Autodesk Inventor part; units mm, degrees
(part 7 of 12)
  line L5353 (-7.555, 11.914) -> (-8.955, 11.914)
  line L5354 (-6.6345, 10.414) -> (-6.5735, 10.414)
  line L5355 (-7.304, 11.914) -> (-7.304, 8.914)
  line L5356 (-7.304, 8.914) -> (-5.904, 8.914)
  line L5357 (-5.904, 8.914) -> (-5.904, 11.914)
  line L5358 (-5.904, 11.914) -> (-7.304, 11.914)
  line L5359 (-10.1295, 25.019) -> (-10.1905, 25.019)
  line L5360 (-9.46, 23.519) -> (-9.46, 26.519)
  line L5361 (-9.46, 26.519) -> (-10.86, 26.519)
  line L5362 (-10.86, 26.519) -> (-10.86, 23.519)
  line L5363 (-10.86, 23.519) -> (-9.46, 23.519)
  line L5364 (-12.065, 6.4465) -> (-12.065, 6.5075)
  line L5365 (-13.565, 5.777) -> (-10.565, 5.777)
  line L5366 (-10.565, 5.777) -> (-10.565, 7.177)
  line L5367 (-10.565, 7.177) -> (-13.565, 7.177)
  line L5368 (-13.565, 7.177) -> (-13.565, 5.777)
  line L5369 (-25.5575, 7.747) -> (-25.4965, 7.747)
  line L5370 (-26.227, 9.247) -> (-26.227, 6.247)
  line L5371 (-26.227, 6.247) -> (-24.827, 6.247)
  line L5372 (-24.827, 6.247) -> (-24.827, 9.247)
  line L5373 (-24.827, 9.247) -> (-26.227, 9.247)
  line L5374 (-25.4965, 25.019) -> (-25.5575, 25.019)
  line L5375 (-24.827, 23.519) -> (-24.827, 26.519)
  line L5376 (-24.827, 26.519) -> (-26.227, 26.519)
  line L5377 (-26.227, 26.519) -> (-26.227, 23.519)
  line L5378 (-26.227, 23.519) -> (-24.827, 23.519)
  line L5379 (-28.8595, 26.797) -> (-28.7985, 26.797)
  line L5380 (-29.529, 28.297) -> (-29.529, 25.297)
  line L5381 (-29.529, 25.297) -> (-28.129, 25.297)
  line L5382 (-28.129, 25.297) -> (-28.129, 28.297)
  line L5383 (-28.129, 28.297) -> (-29.529, 28.297)
  line L5384 (-6.928, 26.273) -> (-6.928, 27.773)
  line L5385 (-6.928, 27.773) -> (-9.328, 27.773)
  line L5386 (-9.328, 27.773) -> (-9.328, 26.273)
  line L5387 (-6.928, 24.273) -> (-6.928, 23.173)
  line L5388 (-6.928, 23.173) -> (-7.328, 22.773)
  line L5389 (-7.328, 22.773) -> (-8.928, 22.773)
  line L5390 (-8.928, 22.773) -> (-9.328, 23.173)
  line L5391 (-9.328, 23.173) -> (-9.328, 24.273)
  line L5392 (-9.144, 24.892) -> (-7.112, 24.892)
  line L5393 (-22.971, 41.967) -> (-24.471, 41.967)
  line L5394 (-24.471, 41.967) -> (-24.471, 39.567)
  line L5395 (-24.471, 39.567) -> (-22.971, 39.567)
  line L5396 (-20.971, 41.967) -> (-19.871, 41.967)
  line L5397 (-19.871, 41.967) -> (-19.471, 41.567)
  line L5398 (-19.471, 41.567) -> (-19.471, 39.967)
  line L5399 (-19.471, 39.967) -> (-19.871, 39.567)
  line L5400 (-19.871, 39.567) -> (-20.971, 39.567)
  line L5401 (-21.59, 39.751) -> (-21.59, 41.783)
  line L5402 (-8.2245, 19.812) -> (-8.2855, 19.812)
  line L5403 (-7.555, 18.312) -> (-7.555, 21.312)
  line L5404 (-7.555, 21.312) -> (-8.955, 21.312)
  line L5405 (-8.955, 21.312) -> (-8.955, 18.312)
  line L5406 (-8.955, 18.312) -> (-7.555, 18.312)
  line L5407 (-17.673, 40.4695) -> (-17.673, 40.5305)
  line L5408 (-19.173, 39.8) -> (-16.173, 39.8)
  line L5409 (-16.173, 39.8) -> (-16.173, 41.2)
  line L5410 (-16.173, 41.2) -> (-19.173, 41.2)
  line L5411 (-19.173, 41.2) -> (-19.173, 39.8)
  line L5412 (-22.0305, 35.9) -> (-21.9695, 35.9)
  line L5413 (-22.7, 37.4) -> (-22.7, 34.4)
  line L5414 (-22.7, 34.4) -> (-21.3, 34.4)
  line L5415 (-21.3, 34.4) -> (-21.3, 37.4)
  line L5416 (-21.3, 37.4) -> (-22.7, 37.4)
  line L5417 (-19.3, 32.0695) -> (-19.3, 32.1305)
  line L5418 (-20.8, 31.4) -> (-17.8, 31.4)
  line L5419 (-17.8, 31.4) -> (-17.8, 32.8)
  line L5420 (-17.8, 32.8) -> (-20.8, 32.8)
  line L5421 (-20.8, 32.8) -> (-20.8, 31.4)
  line L5422 (-22.0305, 32.2) -> (-21.9695, 32.2)
  line L5423 (-22.7, 33.7) -> (-22.7, 30.7)
  line L5424 (-22.7, 30.7) -> (-21.3, 30.7)
  line L5425 (-21.3, 30.7) -> (-21.3, 33.7)
  line L5426 (-21.3, 33.7) -> (-22.7, 33.7)
  line L5427 (-13.7305, 37.6) -> (-13.6695, 37.6)
  line L5428 (-14.4, 39.1) -> (-14.4, 36.1)
  line L5429 (-14.4, 36.1) -> (-13, 36.1)
  line L5430 (-13, 36.1) -> (-13, 39.1)
  line L5431 (-13, 39.1) -> (-14.4, 39.1)
  line L5432 (-12.7, 36.2) -> (-11.3, 36.2)
  line L5433 (-11.3, 36.2) -> (-11.3, 39)
  line L5434 (-11.3, 39) -> (-12.7, 39)
  line L5435 (-12.7, 39) -> (-12.7, 36.2)
  line L5436 (-5.842, 14.0005) -> (-5.842, 13.9395)
  line L5437 (-4.342, 14.67) -> (-7.342, 14.67)
  line L5438 (-7.342, 14.67) -> (-7.342, 13.27)
  line L5439 (-7.342, 13.27) -> (-4.342, 13.27)
  line L5440 (-4.342, 13.27) -> (-4.342, 14.67)
  line L5441 (-5.842, 19.5275) -> (-5.842, 19.5885)
  line L5442 (-7.342, 18.858) -> (-4.342, 18.858)
  line L5443 (-4.342, 18.858) -> (-4.342, 20.258)
  line L5444 (-4.342, 20.258) -> (-7.342, 20.258)
  line L5445 (-7.342, 20.258) -> (-7.342, 18.858)
  line L5446 (-29.3586, 19.8336) -> (-29.3154, 19.7904)
  line L5447 (-28.7713, 21.3676) -> (-30.8926, 19.2463)
  line L5448 (-30.8926, 19.2463) -> (-29.9027, 18.2564)
  line L5449 (-29.9027, 18.2564) -> (-27.7814, 20.3777)
  line L5450 (-27.7814, 20.3777) -> (-28.7713, 21.3676)
  line L5451 (-19.685, 6.4465) -> (-19.685, 6.5075)
  line L5452 (-21.185, 5.777) -> (-18.185, 5.777)
  line L5453 (-18.185, 5.777) -> (-18.185, 7.177)
  line L5454 (-18.185, 7.177) -> (-21.185, 7.177)
  line L5455 (-21.185, 7.177) -> (-21.185, 5.777)
  line L5456 (-18.0086, 3.2766) -> (-18.0086, 4.0894)
  line L5457 (-18.0086, 4.0894) -> (-18.5674, 4.0894)
  line L5458 (-20.8534, 4.0894) -> (-20.8534, 3.2766)
  line L5459 (-20.2946, 4.0894) -> (-20.8534, 4.0894)
  line L5460 (-0.381, 41.148) -> (-0.635, 41.148)
  line L5461 (-5.969, 41.148) -> (-6.223, 41.148)
  circle A419 centre (-3.302, 41.148) radius 2.921
  circle A420 centre (-3.302, 41.148) radius 1.5
  line L5462 (-35.179, 41.148) -> (-34.925, 41.148)
  line L5463 (-29.591, 41.148) -> (-29.337, 41.148)
  circle A421 centre (-32.258, 41.148) radius 2.921
  circle A422 centre (-32.258, 41.148) radius 1.5
  line L5464 (-35.179, 4.699) -> (-35.179, 3.429)
  line L5465 (-35.179, 3.429) -> (-34.544, 2.794)
  line L5466 (-34.544, 2.794) -> (-33.274, 2.794)
  line L5467 (-33.274, 2.794) -> (-32.639, 3.429)
  line L5468 (-34.544, 7.874) -> (-35.179, 7.239)
  line L5469 (-35.179, 7.239) -> (-35.179, 5.969)
  line L5470 (-35.179, 5.969) -> (-34.544, 5.334)
  line L5471 (-34.544, 5.334) -> (-33.274, 5.334)
  line L5472 (-33.274, 5.334) -> (-32.639, 5.969)
  line L5473 (-32.639, 5.969) -> (-32.639, 7.239)
  line L5474 (-32.639, 7.239) -> (-33.274, 7.874)
  line L5475 (-35.179, 4.699) -> (-34.544, 5.334)
  line L5476 (-33.274, 5.334) -> (-32.639, 4.699)
  line L5477 (-32.639, 3.429) -> (-32.639, 4.699)
  line L5478 (-35.179, 12.319) -> (-35.179, 11.049)
  line L5479 (-35.179, 11.049) -> (-34.544, 10.414)
  line L5480 (-34.544, 10.414) -> (-33.274, 10.414)
  line L5481 (-33.274, 10.414) -> (-32.639, 11.049)
  line L5482 (-34.544, 10.414) -> (-35.179, 9.779)
  line L5483 (-35.179, 9.779) -> (-35.179, 8.509)
  line L5484 (-35.179, 8.509) -> (-34.544, 7.874)
  line L5485 (-34.544, 7.874) -> (-33.274, 7.874)
  line L5486 (-33.274, 7.874) -> (-32.639, 8.509)
  line L5487 (-32.639, 8.509) -> (-32.639, 9.779)
  line L5488 (-32.639, 9.779) -> (-33.274, 10.414)
  line L5489 (-34.544, 15.494) -> (-35.179, 14.859)
  line L5490 (-35.179, 14.859) -> (-35.179, 13.589)
  line L5491 (-35.179, 13.589) -> (-34.544, 12.954)
  line L5492 (-34.544, 12.954) -> (-33.274, 12.954)
  line L5493 (-33.274, 12.954) -> (-32.639, 13.589)
  line L5494 (-32.639, 13.589) -> (-32.639, 14.859)
  line L5495 (-32.639, 14.859) -> (-33.274, 15.494)
  line L5496 (-35.179, 12.319) -> (-34.544, 12.954)
  line L5497 (-33.274, 12.954) -> (-32.639, 12.319)
  line L5498 (-32.639, 11.049) -> (-32.639, 12.319)
  line L5499 (-35.179, 19.939) -> (-35.179, 18.669)
  line L5500 (-35.179, 18.669) -> (-34.544, 18.034)
  line L5501 (-34.544, 18.034) -> (-33.274, 18.034)
  line L5502 (-33.274, 18.034) -> (-32.639, 18.669)
  line L5503 (-34.544, 18.034) -> (-35.179, 17.399)
  line L5504 (-35.179, 17.399) -> (-35.179, 16.129)
  line L5505 (-35.179, 16.129) -> (-34.544, 15.494)
  line L5506 (-34.544, 15.494) -> (-33.274, 15.494)
  line L5507 (-33.274, 15.494) -> (-32.639, 16.129)
  line L5508 (-32.639, 16.129) -> (-32.639, 17.399)
  line L5509 (-32.639, 17.399) -> (-33.274, 18.034)
  line L5510 (-34.544, 20.574) -> (-33.274, 20.574)
  line L5511 (-35.179, 19.939) -> (-34.544, 20.574)
  line L5512 (-33.274, 20.574) -> (-32.639, 19.939)
  line L5513 (-32.639, 18.669) -> (-32.639, 19.939)
  line L5514 (-35.179, 2.159) -> (-35.179, 0.889)
  line L5515 (-35.179, 0.889) -> (-34.544, 0.254)
  line L5516 (-34.544, 0.254) -> (-33.274, 0.254)
  line L5517 (-33.274, 0.254) -> (-32.639, 0.889)
  line L5518 (-35.179, 2.159) -> (-34.544, 2.794)
  line L5519 (-33.274, 2.794) -> (-32.639, 2.159)
  line L5520 (-32.639, 0.889) -> (-32.639, 2.159)
  line L5521 (-2.921, 4.699) -> (-2.921, 3.429)
  line L5522 (-2.921, 3.429) -> (-2.286, 2.794)
  line L5523 (-2.286, 2.794) -> (-1.016, 2.794)
  line L5524 (-1.016, 2.794) -> (-0.381, 3.429)
  line L5525 (-2.286, 7.874) -> (-2.921, 7.239)
  line L5526 (-2.921, 7.239) -> (-2.921, 5.969)
  line L5527 (-2.921, 5.969) -> (-2.286, 5.334)
  line L5528 (-2.286, 5.334) -> (-1.016, 5.334)
  line L5529 (-1.016, 5.334) -> (-0.381, 5.969)
  line L5530 (-0.381, 5.969) -> (-0.381, 7.239)
  line L5531 (-0.381, 7.239) -> (-1.016, 7.874)
  line L5532 (-2.921, 4.699) -> (-2.286, 5.334)
  line L5533 (-1.016, 5.334) -> (-0.381, 4.699)
  line L5534 (-0.381, 3.429) -> (-0.381, 4.699)
  line L5535 (-2.921, 12.319) -> (-2.921, 11.049)
  line L5536 (-2.921, 11.049) -> (-2.286, 10.414)
  line L5537 (-2.286, 10.414) -> (-1.016, 10.414)
  line L5538 (-1.016, 10.414) -> (-0.381, 11.049)
  line L5539 (-2.286, 10.414) -> (-2.921, 9.779)
  line L5540 (-2.921, 9.779) -> (-2.921, 8.509)
  line L5541 (-2.921, 8.509) -> (-2.286, 7.874)
  line L5542 (-2.286, 7.874) -> (-1.016, 7.874)
  line L5543 (-1.016, 7.874) -> (-0.381, 8.509)
  line L5544 (-0.381, 8.509) -> (-0.381, 9.779)
  line L5545 (-0.381, 9.779) -> (-1.016, 10.414)
  line L5546 (-2.286, 15.494) -> (-2.921, 14.859)
  line L5547 (-2.921, 14.859) -> (-2.921, 13.589)
  line L5548 (-2.921, 13.589) -> (-2.286, 12.954)
  line L5549 (-2.286, 12.954) -> (-1.016, 12.954)
  line L5550 (-1.016, 12.954) -> (-0.381, 13.589)
  line L5551 (-0.381, 13.589) -> (-0.381, 14.859)
  line L5552 (-0.381, 14.859) -> (-1.016, 15.494)
  line L5553 (-2.921, 12.319) -> (-2.286, 12.954)
  line L5554 (-1.016, 12.954) -> (-0.381, 12.319)
  line L5555 (-0.381, 11.049) -> (-0.381, 12.319)
  line L5556 (-2.921, 19.939) -> (-2.921, 18.669)
  line L5557 (-2.921, 18.669) -> (-2.286, 18.034)
  line L5558 (-2.286, 18.034) -> (-1.016, 18.034)
  line L5559 (-1.016, 18.034) -> (-0.381, 18.669)
  line L5560 (-2.286, 18.034) -> (-2.921, 17.399)
  line L5561 (-2.921, 17.399) -> (-2.921, 16.129)
  line L5562 (-2.921, 16.129) -> (-2.286, 15.494)
  line L5563 (-2.286, 15.494) -> (-1.016, 15.494)
  line L5564 (-1.016, 15.494) -> (-0.381, 16.129)
  line L5565 (-0.381, 16.129) -> (-0.381, 17.399)
  line L5566 (-0.381, 17.399) -> (-1.016, 18.034)
  line L5567 (-2.286, 20.574) -> (-1.016, 20.574)
  line L5568 (-2.921, 19.939) -> (-2.286, 20.574)
  line L5569 (-1.016, 20.574) -> (-0.381, 19.939)
  line L5570 (-0.381, 18.669) -> (-0.381, 19.939)
  line L5571 (-2.921, 2.159) -> (-2.921, 0.889)
  line L5572 (-2.921, 0.889) -> (-2.286, 0.254)
  line L5573 (-2.286, 0.254) -> (-1.016, 0.254)
  line L5574 (-1.016, 0.254) -> (-0.381, 0.889)
  line L5575 (-2.921, 2.159) -> (-2.286, 2.794)
  line L5576 (-1.016, 2.794) -> (-0.381, 2.159)
  line L5577 (-0.381, 0.889) -> (-0.381, 2.159)
  line L5578 (-31.369, 9.779) -> (-31.369, 8.509)
  line L5579 (-31.369, 8.509) -> (-30.734, 7.874)
  line L5580 (-30.734, 7.874) -> (-29.464, 7.874)
  line L5581 (-29.464, 7.874) -> (-28.829, 8.509)
  line L5582 (-30.734, 12.954) -> (-31.369, 12.319)
  line L5583 (-31.369, 12.319) -> (-31.369, 11.049)
  line L5584 (-31.369, 11.049) -> (-30.734, 10.414)
  line L5585 (-30.734, 10.414) -> (-29.464, 10.414)
  line L5586 (-29.464, 10.414) -> (-28.829, 11.049)
  line L5587 (-28.829, 11.049) -> (-28.829, 12.319)
  line L5588 (-28.829, 12.319) -> (-29.464, 12.954)
  line L5589 (-31.369, 9.779) -> (-30.734, 10.414)
  line L5590 (-29.464, 10.414) -> (-28.829, 9.779)
  line L5591 (-28.829, 8.509) -> (-28.829, 9.779)
  line L5592 (-31.369, 17.399) -> (-31.369, 16.129)
  line L5593 (-31.369, 16.129) -> (-30.734, 15.494)
  line L5594 (-30.734, 15.494) -> (-29.464, 15.494)
  line L5595 (-29.464, 15.494) -> (-28.829, 16.129)
  line L5596 (-30.734, 15.494) -> (-31.369, 14.859)
  line L5597 (-31.369, 14.859) -> (-31.369, 13.589)
  line L5598 (-31.369, 13.589) -> (-30.734, 12.954)
  line L5599 (-30.734, 12.954) -> (-29.464, 12.954)
  line L5600 (-29.464, 12.954) -> (-28.829, 13.589)
  line L5601 (-28.829, 13.589) -> (-28.829, 14.859)
  line L5602 (-28.829, 14.859) -> (-29.464, 15.494)
  line L5603 (-30.734, 18.034) -> (-29.464, 18.034)
  line L5604 (-31.369, 17.399) -> (-30.734, 18.034)
  line L5605 (-29.464, 18.034) -> (-28.829, 17.399)
  line L5606 (-28.829, 16.129) -> (-28.829, 17.399)
  line L5607 (-31.369, 7.239) -> (-31.369, 5.969)
  line L5608 (-31.369, 5.969) -> (-30.734, 5.334)
  line L5609 (-30.734, 5.334) -> (-29.464, 5.334)
  line L5610 (-29.464, 5.334) -> (-28.829, 5.969)
  line L5611 (-31.369, 7.239) -> (-30.734, 7.874)
  line L5612 (-29.464, 7.874) -> (-28.829, 7.239)
  line L5613 (-28.829, 5.969) -> (-28.829, 7.239)
  line L5614 (-5.653, 11.914) -> (-5.653, 8.914)
  line L5615 (-5.653, 8.914) -> (-4.253, 8.914)
  line L5616 (-4.253, 8.914) -> (-4.253, 11.914)
  line L5617 (-4.253, 11.914) -> (-5.653, 11.914)
  line L5618 (-24.487, 5.777) -> (-21.487, 5.777)
  line L5619 (-21.487, 5.777) -> (-21.487, 7.177)
  line L5620 (-21.487, 7.177) -> (-24.487, 7.177)
  line L5621 (-24.487, 7.177) -> (-24.487, 5.777)
  line L5622 (-1.24, 31.399) -> (-0.94, 31.399)
  line L5623 (-0.94, 31.399) -> (-0.94, 28.799)
  line L5624 (-0.94, 28.799) -> (-1.24, 28.799)
  line L5625 (-3.84, 31.399) -> (-4.14, 31.399)
  line L5626 (-4.14, 31.399) -> (-4.14, 28.799)
  line L5627 (-4.14, 28.799) -> (-3.84, 28.799)
  line L5628 (-3.94, 31.899) -> (-3.94, 32.499)
  line L5629 (-3.94, 32.499) -> (-3.34, 32.499)
  line L5630 (-33.1614, 34.4142) -> (-33.5857, 33.9899)
  line L5631 (-33.5857, 33.9899) -> (-34.7171, 35.1213)
  line L5632 (-34.7171, 35.1213) -> (-34.2928, 35.5456)
  line L5633 (-31.7472, 35.8284) -> (-31.3229, 36.2527)
  line L5634 (-31.3229, 36.2527) -> (-32.4543, 37.3841)
  line L5635 (-32.4543, 37.3841) -> (-32.8786, 36.9598)
  line L5636 (-32.3129, 35.4042) -> (-32.8079, 35.8991)
  line L5637 (-32.8079, 35.8991) -> (-33.3028, 36.3941)
  line L5638 (-32.8079, 35.8991) -> (-32.8079, 35.0506)
  line L5639 (-32.8079, 35.0506) -> (-33.6564, 35.8991)
  line L5640 (-33.6564, 35.8991) -> (-32.8079, 35.8991)
  line L5641 (-3.8128, 35.8284) -> (-4.2371, 36.2527)
  line L5642 (-4.2371, 36.2527) -> (-3.1057, 37.3841)
  line L5643 (-3.1057, 37.3841) -> (-2.6814, 36.9598)
  line L5644 (-2.3986, 34.4142) -> (-1.9743, 33.9899)
  line L5645 (-1.9743, 33.9899) -> (-0.8429, 35.1213)
  line L5646 (-0.8429, 35.1213) -> (-1.2672, 35.5456)
  line L5647 (-2.8228, 34.9799) -> (-2.3279, 35.4749)
  line L5648 (-2.3279, 35.4749) -> (-1.8329, 35.9698)
  line L5649 (-2.3279, 35.4749) -> (-3.1764, 35.4749)
  line L5650 (-3.1764, 35.4749) -> (-2.3279, 36.3234)
  line L5651 (-2.3279, 36.3234) -> (-2.3279, 35.4749)
  line L5652 (-9.78, 28.068) -> (-9.78, 34.091)
  line L5653 (-9.78, 34.091) -> (-9.78, 38.045)
  line L5654 (-9.78, 38.045) -> (-9.78, 44.068)
  line L5655 (-9.78, 44.068) -> (-25.78, 44.068)
  line L5656 (-25.78, 44.068) -> (-25.78, 38.045)
  line L5657 (-25.78, 38.045) -> (-25.78, 34.091)
  line L5658 (-25.78, 34.091) -> (-25.78, 28.068)
  line L5659 (-25.78, 28.068) -> (-9.78, 28.068)
  arc A423 (-9.78, 34.091) -> (-9.78, 38.045) centre (-7.803, 36.068) ccw
  arc A424 (-25.78, 38.045) -> (-25.78, 34.091) centre (-27.757, 36.068) ccw
  line L5660 (-10.78, 29.068) -> (-24.78, 29.068)
  line L5661 (-24.78, 29.068) -> (-24.78, 43.068)
  line L5662 (-24.78, 43.068) -> (-10.78, 43.068)
  line L5663 (-10.78, 43.068) -> (-10.78, 29.068)
  line L5664 (-27.051, 40.005) -> (-26.67, 39.878)
  line L5665 (-26.67, 39.878) -> (-26.543, 40.005)
  line L5666 (-26.543, 40.005) -> (-26.797, 40.386)
  line L5667 (-26.797, 40.386) -> (-26.543, 40.767)
  line L5668 (-26.543, 40.767) -> (-26.289, 40.767)
  line L5669 (-26.289, 40.767) -> (-26.289, 41.021)
  line L5670 (-26.289, 41.021) -> (-26.67, 41.021)
  line L5671 (-26.67, 41.021) -> (-26.797, 41.402)
  line L5672 (-26.797, 41.402) -> (-26.543, 41.783)
  line L5673 (-26.543, 41.783) -> (-26.67, 41.91)
  line L5674 (-26.67, 41.91) -> (-27.051, 41.656)
  line L5675 (-27.051, 41.656) -> (-27.432, 41.91)
  line L5676 (-27.432, 41.91) -> (-27.432, 42.164)
  line L5677 (-27.432, 42.164) -> (-27.686, 42.164)
  line L5678 (-27.686, 42.164) -> (-27.813, 41.783)
  line L5679 (-27.813, 41.783) -> (-28.194, 41.656)
  line L5680 (-28.194, 41.656) -> (-28.448, 41.91)
  line L5681 (-28.448, 41.91) -> (-28.575, 41.783)
  line L5682 (-28.575, 41.783) -> (-28.448, 41.402)
  line L5683 (-28.448, 41.402) -> (-28.575, 41.021)
  line L5684 (-28.575, 41.021) -> (-28.956, 41.021)
  line L5685 (-28.956, 41.021) -> (-28.829, 40.767)
  line L5686 (-28.829, 40.767) -> (-28.448, 40.64)
  line L5687 (-28.448, 40.64) -> (-28.448, 40.259)
  line L5688 (-28.448, 40.259) -> (-28.575, 40.005)
  line L5689 (-28.575, 40.005) -> (-28.448, 39.878)
  line L5690 (-28.448, 39.878) -> (-28.194, 40.005)
  line L5691 (-28.194, 40.005) -> (-28.067, 40.005)
  line L5692 (-28.067, 40.005) -> (-27.94, 40.386)
  line L5693 (-27.94, 40.386) -> (-28.194, 40.894)
  line L5694 (-28.194, 40.894) -> (-27.94, 41.275)
  line L5695 (-27.94, 41.275) -> (-27.559, 41.402)
  line L5696 (-27.559, 41.402) -> (-27.178, 41.275)
  line L5697 (-27.178, 41.275) -> (-27.051, 40.894)
  line L5698 (-27.051, 40.894) -> (-27.178, 40.513)
  line L5699 (-27.178, 40.513) -> (-27.305, 40.386)
  line L5700 (-27.305, 40.386) -> (-27.051, 40.005)
  line L5701 (-26.6192, 39.9288) -> (-26.8224, 39.9288)
  line L5702 (-28.3464, 39.9288) -> (-28.4988, 39.9288)
  line L5703 (-26.5938, 40.0812) -> (-27.1018, 40.0812)
  line L5704 (-28.0416, 40.0812) -> (-28.5369, 40.0812)
  line L5705 (-26.6954, 40.2336) -> (-27.2034, 40.2336)
  line L5706 (-27.9908, 40.2336) -> (-28.4607, 40.2336)
  line L5707 (-26.797, 40.386) -> (-27.305, 40.386)
  line L5708 (-27.94, 40.386) -> (-28.448, 40.386)
  line L5709 (-26.6954, 40.5384) -> (-27.1695, 40.5384)
  line L5710 (-28.0162, 40.5384) -> (-28.448, 40.5384)
  line L5711 (-26.5938, 40.6908) -> (-27.1187, 40.6908)
  line L5712 (-28.0924, 40.6908) -> (-28.6004, 40.6908)
  line L5713 (-26.289, 40.8432) -> (-27.0679, 40.8432)
  line L5714 (-28.1686, 40.8432) -> (-28.8671, 40.8432)
  line L5715 (-26.289, 40.9956) -> (-27.0849, 40.9956)
  line L5716 (-28.1263, 40.9956) -> (-28.9433, 40.9956)
  line L5717 (-26.7123, 41.148) -> (-27.1357, 41.148)
  line L5718 (-28.0247, 41.148) -> (-28.5327, 41.148)
  line L5719 (-26.7631, 41.3004) -> (-27.2542, 41.3004)
  line L5720 (-27.8638, 41.3004) -> (-28.4819, 41.3004)
  line L5721 (-26.7631, 41.4528) -> (-28.4649, 41.4528)
  line L5722 (-26.6615, 41.6052) -> (-28.5157, 41.6052)
  line L5723 (-26.5599, 41.7576) -> (-26.8986, 41.7576)
  line L5724 (-27.2034, 41.7576) -> (-27.8892, 41.7576)
  line L5725 (-28.2956, 41.7576) -> (-28.5665, 41.7576)
  line L5726 (-27.432, 41.91) -> (-27.7707, 41.91)
  line L5727 (-27.432, 42.0624) -> (-27.7199, 42.0624)
  line L5728 (-27.3812, 40.4622) -> (-27.1272, 39.878)
  line L5729 (-27.1272, 39.878) -> (-27.0002, 39.9542)
  line L5730 (-27.0002, 39.9542) -> (-26.6954, 39.751)
  line L5731 (-26.6954, 39.751) -> (-26.4668, 39.9796)
  line L5732 (-26.4668, 39.9796) -> (-26.67, 40.3098)
  line L5733 (-26.67, 40.3098) -> (-26.543, 40.64)
  line L5734 (-26.543, 40.64) -> (-26.162, 40.7162)
  line L5735 (-26.162, 40.7162) -> (-26.162, 41.0464)
  line L5736 (-26.162, 41.0464) -> (-26.543, 41.0972)
  line L5737 (-26.543, 41.0972) -> (-26.6954, 41.4274)
  line L5738 (-26.6954, 41.4274) -> (-26.4668, 41.7576)
  line L5739 (-26.4668, 41.7576) -> (-26.6954, 41.9862)
  line L5740 (-26.6954, 41.9862) -> (-27.0256, 41.7576)
  line L5741 (-27.0256, 41.7576) -> (-27.3304, 41.8846)
  line L5742 (-27.3304, 41.8846) -> (-27.4066, 42.291)
  line L5743 (-27.4066, 42.291) -> (-27.7368, 42.291)
  line L5744 (-27.7368, 42.291) -> (-27.813, 41.8846)
  line L5745 (-27.813, 41.8846) -> (-28.1178, 41.7576)
  line L5746 (-28.1178, 41.7576) -> (-28.4734, 41.9862)
  line L5747 (-28.4734, 41.9862) -> (-28.702, 41.7576)
  line L5748 (-28.702, 41.7576) -> (-28.4734, 41.4274)
  line L5749 (-28.4734, 41.4274) -> (-28.6004, 41.1226)
  line L5750 (-28.6004, 41.1226) -> (-28.9814, 41.0464)
  line L5751 (-28.9814, 41.0464) -> (-28.9814, 40.7162)
  line L5752 (-28.9814, 40.7162) -> (-28.6258, 40.64)
  line L5753 (-28.6258, 40.64) -> (-28.4734, 40.3098)
  line L5754 (-28.4734, 40.3098) -> (-28.702, 39.9796)
  line L5755 (-28.702, 39.9796) -> (-28.4734, 39.751)
  line L5756 (-28.4734, 39.751) -> (-28.1686, 39.9542)
  line L5757 (-28.1686, 39.9542) -> (-28.0162, 39.878)
  line L5758 (-28.0162, 39.878) -> (-27.7876, 40.4622)
  arc A425 (-27.3812, 40.4622) -> (-27.7876, 40.4622) centre (-27.5844, 40.8686) ccw
  line L5759 (-2.756, 25.719) -> (-2.156, 25.719)
  line L5760 (-2.156, 25.719) -> (-2.156, 24.919)
  line L5761 (-4.356, 25.719) -> (-4.956, 25.719)
  line L5762 (-4.956, 25.719) -> (-4.956, 24.919)
  line L5763 (-6.669, 26.519) -> (-6.669, 23.519)
  line L5764 (-6.669, 23.519) -> (-5.269, 23.519)
  line L5765 (-5.269, 23.519) -> (-5.269, 26.519)
  line L5766 (-5.269, 26.519) -> (-6.669, 26.519)
  line L5767 (-1.843, 26.519) -> (-1.843, 23.519)
  line L5768 (-1.843, 23.519) -> (-0.443, 23.519)
  line L5769 (-0.443, 23.519) -> (-0.443, 26.519)
  line L5770 (-0.443, 26.519) -> (-1.843, 26.519)
  line L5771 (-20.804, 29.399) -> (-17.804, 29.399)
  line L5772 (-17.804, 29.399) -> (-17.804, 30.799)
  line L5773 (-17.804, 30.799) -> (-20.804, 30.799)
  line L5774 (-20.804, 30.799) -> (-20.804, 29.399)
  line L5775 (-24.4, 33.7) -> (-24.4, 30.7)
  line L5776 (-24.4, 30.7) -> (-23, 30.7)
  line L5777 (-23, 30.7) -> (-23, 33.7)
  line L5778 (-23, 33.7) -> (-24.4, 33.7)
  line L5779 (-7.1635, 28.803) -> (-5.6635, 28.803)
  line L5780 (-5.6635, 31.903) -> (-7.1635, 31.903)
  line L5781 (-28.817, 21.691) -> (-27.317, 21.691)
  line L5782 (-27.317, 24.791) -> (-28.817, 24.791)
  line L5783 (-28.817, 29.184) -> (-27.317, 29.184)
  line L5784 (-27.317, 32.284) -> (-28.817, 32.284)
  line L5785 (-15.35, 32.35) -> (-15.35, 30.85)
  line L5786 (-13.85, 30.85) -> (-13.85, 32.35)
  line L5787 (-11.38, 9.483) -> (-24.18, 9.483)
  line L5788 (-24.68, 9.983) -> (-24.68, 22.783)
  line L5789 (-24.18, 23.283) -> (-11.38, 23.283)
  line L5790 (-11.38, 23.283) -> (-10.88, 22.783)
  line L5791 (-10.88, 22.783) -> (-10.88, 9.983)
  line L5792 (-24.18, 23.283) -> (-24.68, 22.783)
  line L5793 (-24.18, 9.483) -> (-24.68, 9.983)
  line L5794 (-11.38, 9.483) -> (-10.88, 9.983)
  circle A426 centre (-11.88, 22.283) radius 0.5
  line L5795 (-20.575, 33.775) -> (-15.225, 33.775)
  line L5796 (-15.225, 33.775) -> (-15.225, 39.025)
  line L5797 (-15.225, 39.025) -> (-20.575, 39.025)
  line L5798 (-20.575, 39.025) -> (-20.575, 33.775)
  line L5799 (-13.203, 0.394) -> (-9.403, 0.394)
  line L5800 (-9.403, 0.394) -> (-9.403, 5.194)
  line L5801 (-9.403, 5.194) -> (-13.203, 5.194)
  line L5802 (-13.203, 5.194) -> (-13.203, 0.394)
  circle A427 centre (-9.903, 4.694) radius 0.15
  line L5803 (-35.466, 20.943) -> (-35.466, 32.943)
  line L5804 (-35.466, 32.943) -> (-29.866, 32.943)
  line L5805 (-29.866, 32.943) -> (-29.866, 20.943)
  line L5806 (-29.866, 20.943) -> (-35.466, 20.943)
  line L5807 (-22.09, 0.0025) -> (-31.25, 0.0025)
  line L5808 (-22.09, 0.0025) -> (-22.09, 5.1575)
  line L5809 (-22.09, 5.1575) -> (-31.25, 5.1575)
  line L5810 (-31.25, 5.1575) -> (-31.25, 0.0025)
  line L5811 (-7.388, 17.402) -> (-7.388, 16.202)
  line L5812 (-6.238, 15.152) -> (-5.638, 15.152)
  line L5813 (-4.488, 16.202) -> (-4.488, 17.402)
  line L5814 (-6.288, 18.402) -> (-5.688, 18.402)
  circle A428 centre (-4.519, 18.414) radius 0.1
  line L5815 (-26.678, 28.197) -> (-26.678, 27.197)
  line L5816 (-26.678, 27.197) -> (-27.678, 27.197)
  line L5817 (-27.678, 27.197) -> (-27.678, 28.197)
  line L5818 (-27.678, 28.197) -> (-26.678, 28.197)
  line L5819 (-26.678, 26.397) -> (-26.678, 25.397)
  line L5820 (-26.678, 25.397) -> (-27.678, 25.397)
  line L5821 (-27.678, 25.397) -> (-27.678, 26.397)
  line L5822 (-27.678, 26.397) -> (-26.678, 26.397)
  line L5823 (-16.01, 4.702) -> (-16.01, 3.702)
  line L5824 (-16.01, 3.702) -> (-17.01, 3.702)
  line L5825 (-17.01, 3.702) -> (-17.01, 4.702)
  line L5826 (-17.01, 4.702) -> (-16.01, 4.702)
  line L5827 (-16.01, 2.902) -> (-16.01, 1.902)
  line L5828 (-16.01, 1.902) -> (-17.01, 1.902)
  line L5829 (-17.01, 1.902) -> (-17.01, 2.902)
  line L5830 (-17.01, 2.902) -> (-16.01, 2.902)
  line L5831 (-6.723, 4.821) -> (-5.723, 4.821)
  line L5832 (-5.723, 4.821) -> (-5.723, 3.821)
  line L5833 (-5.723, 3.821) -> (-6.723, 3.821)
  line L5834 (-6.723, 3.821) -> (-6.723, 4.821)
  line L5835 (-6.723, 2.021) -> (-5.723, 2.021)
  line L5836 (-5.723, 2.021) -> (-5.723, 1.021)
  line L5837 (-5.723, 1.021) -> (-6.723, 1.021)
  line L5838 (-6.723, 1.021) -> (-6.723, 2.021)
  line L5839 (-7.755, 11.714) -> (-7.755, 10.714)
  line L5840 (-7.755, 10.714) -> (-8.755, 10.714)
  line L5841 (-8.755, 10.714) -> (-8.755, 11.714)
  line L5842 (-8.755, 11.714) -> (-7.755, 11.714)
  line L5843 (-7.755, 10.114) -> (-7.755, 9.114)
  line L5844 (-7.755, 9.114) -> (-8.755, 9.114)
  line L5845 (-8.755, 9.114) -> (-8.755, 10.114)
  line L5846 (-8.755, 10.114) -> (-7.755, 10.114)
  line L5847 (-6.104, 11.714) -> (-6.104, 10.714)
  line L5848 (-6.104, 10.714) -> (-7.104, 10.714)
  line L5849 (-7.104, 10.714) -> (-7.104, 11.714)
  line L5850 (-7.104, 11.714) -> (-6.104, 11.714)
  line L5851 (-6.104, 10.114) -> (-6.104, 9.114)
  line L5852 (-6.104, 9.114) -> (-7.104, 9.114)
  line L5853 (-7.104, 9.114) -> (-7.104, 10.114)
  line L5854 (-7.104, 10.114) -> (-6.104, 10.114)
  line L5855 (-10.66, 23.719) -> (-10.66, 24.719)
  line L5856 (-10.66, 24.719) -> (-9.66, 24.719)
  line L5857 (-9.66, 24.719) -> (-9.66, 23.719)
  line L5858 (-9.66, 23.719) -> (-10.66, 23.719)
  line L5859 (-10.66, 25.319) -> (-10.66, 26.319)
  line L5860 (-10.66, 26.319) -> (-9.66, 26.319)
  line L5861 (-9.66, 26.319) -> (-9.66, 25.319)
  line L5862 (-9.66, 25.319) -> (-10.66, 25.319)
  line L5863 (-13.365, 6.977) -> (-12.365, 6.977)
  line L5864 (-12.365, 6.977) -> (-12.365, 5.977)
  line L5865 (-12.365, 5.977) -> (-13.365, 5.977)
  line L5866 (-13.365, 5.977) -> (-13.365, 6.977)
  line L5867 (-11.765, 6.977) -> (-10.765, 6.977)
  line L5868 (-10.765, 6.977) -> (-10.765, 5.977)
  line L5869 (-10.765, 5.977) -> (-11.765, 5.977)
  line L5870 (-11.765, 5.977) -> (-11.765, 6.977)
  line L5871 (-25.027, 9.047) -> (-25.027, 8.047)
  line L5872 (-25.027, 8.047) -> (-26.027, 8.047)
  line L5873 (-26.027, 8.047) -> (-26.027, 9.047)
  line L5874 (-26.027, 9.047) -> (-25.027, 9.047)
  line L5875 (-25.027, 7.447) -> (-25.027, 6.447)
  line L5876 (-25.027, 6.447) -> (-26.027, 6.447)
  line L5877 (-26.027, 6.447) -> (-26.027, 7.447)
  line L5878 (-26.027, 7.447) -> (-25.027, 7.447)
  line L5879 (-26.027, 23.719) -> (-26.027, 24.719)
  line L5880 (-26.027, 24.719) -> (-25.027, 24.719)
  line L5881 (-25.027, 24.719) -> (-25.027, 23.719)
  line L5882 (-25.027, 23.719) -> (-26.027, 23.719)
  line L5883 (-26.027, 25.319) -> (-26.027, 26.319)
  line L5884 (-26.027, 26.319) -> (-25.027, 26.319)
  line L5885 (-25.027, 26.319) -> (-25.027, 25.319)
  line L5886 (-25.027, 25.319) -> (-26.027, 25.319)
  line L5887 (-28.329, 28.097) -> (-28.329, 27.097)
  line L5888 (-28.329, 27.097) -> (-29.329, 27.097)
  line L5889 (-29.329, 27.097) -> (-29.329, 28.097)
  line L5890 (-29.329, 28.097) -> (-28.329, 28.097)
  line L5891 (-28.329, 26.497) -> (-28.329, 25.497)
  line L5892 (-28.329, 25.497) -> (-29.329, 25.497)
  line L5893 (-29.329, 25.497) -> (-29.329, 26.497)
  line L5894 (-29.329, 26.497) -> (-28.329, 26.497)
  line L5895 (-7.628, 23.373) -> (-8.628, 23.373)
  line L5896 (-8.628, 23.373) -> (-8.628, 24.373)
  line L5897 (-8.628, 24.373) -> (-7.628, 24.373)
  line L5898 (-7.628, 24.373) -> (-7.628, 23.373)
  line L5899 (-7.628, 26.173) -> (-8.628, 26.173)
  line L5900 (-8.628, 26.173) -> (-8.628, 27.173)
  line L5901 (-8.628, 27.173) -> (-7.628, 27.173)
  line L5902 (-7.628, 27.173) -> (-7.628, 26.173)
  line L5903 (-20.071, 41.267) -> (-20.071, 40.267)
  line L5904 (-20.071, 40.267) -> (-21.071, 40.267)
  line L5905 (-21.071, 40.267) -> (-21.071, 41.267)
  line L5906 (-21.071, 41.267) -> (-20.071, 41.267)
  line L5907 (-22.871, 41.267) -> (-22.871, 40.267)
  line L5908 (-22.871, 40.267) -> (-23.871, 40.267)
  line L5909 (-23.871, 40.267) -> (-23.871, 41.267)
  line L5910 (-23.871, 41.267) -> (-22.871, 41.267)
  line L5911 (-8.755, 18.512) -> (-8.755, 19.512)
  line L5912 (-8.755, 19.512) -> (-7.755, 19.512)
  line L5913 (-7.755, 19.512) -> (-7.755, 18.512)
  line L5914 (-7.755, 18.512) -> (-8.755, 18.512)
  line L5915 (-8.755, 20.112) -> (-8.755, 21.112)
  line L5916 (-8.755, 21.112) -> (-7.755, 21.112)
  line L5917 (-7.755, 21.112) -> (-7.755, 20.112)
  line L5918 (-7.755, 20.112) -> (-8.755, 20.112)
  line L5919 (-18.973, 41) -> (-17.973, 41)
  line L5920 (-17.973, 41) -> (-17.973, 40)
  line L5921 (-17.973, 40) -> (-18.973, 40)
  line L5922 (-18.973, 40) -> (-18.973, 41)
  line L5923 (-17.373, 41) -> (-16.373, 41)
  line L5924 (-16.373, 41) -> (-16.373, 40)
  line L5925 (-16.373, 40) -> (-17.373, 40)
  line L5926 (-17.373, 40) -> (-17.373, 41)
  line L5927 (-21.5, 37.2) -> (-21.5, 36.2)
  line L5928 (-21.5, 36.2) -> (-22.5, 36.2)
  line L5929 (-22.5, 36.2) -> (-22.5, 37.2)
  line L5930 (-22.5, 37.2) -> (-21.5, 37.2)
  line L5931 (-21.5, 35.6) -> (-21.5, 34.6)
  line L5932 (-21.5, 34.6) -> (-22.5, 34.6)
  line L5933 (-22.5, 34.6) -> (-22.5, 35.6)
  line L5934 (-22.5, 35.6) -> (-21.5, 35.6)
  line L5935 (-20.6, 32.6) -> (-19.6, 32.6)
  line L5936 (-19.6, 32.6) -> (-19.6, 31.6)
  line L5937 (-19.6, 31.6) -> (-20.6, 31.6)
  line L5938 (-20.6, 31.6) -> (-20.6, 32.6)
  line L5939 (-19, 32.6) -> (-18, 32.6)
  line L5940 (-18, 32.6) -> (-18, 31.6)
  line L5941 (-18, 31.6) -> (-19, 31.6)
  line L5942 (-19, 31.6) -> (-19, 32.6)
  line L5943 (-21.5, 33.5) -> (-21.5, 32.5)
  line L5944 (-21.5, 32.5) -> (-22.5, 32.5)
  line L5945 (-22.5, 32.5) -> (-22.5, 33.5)
  line L5946 (-22.5, 33.5) -> (-21.5, 33.5)
  line L5947 (-21.5, 31.9) -> (-21.5, 30.9)
  line L5948 (-21.5, 30.9) -> (-22.5, 30.9)
  line L5949 (-22.5, 30.9) -> (-22.5, 31.9)
  line L5950 (-22.5, 31.9) -> (-21.5, 31.9)
  line L5951 (-13.2, 38.9) -> (-13.2, 37.9)
  line L5952 (-13.2, 37.9) -> (-14.2, 37.9)
  line L5953 (-14.2, 37.9) -> (-14.2, 38.9)
  line L5954 (-14.2, 38.9) -> (-13.2, 38.9)
  line L5955 (-13.2, 37.3) -> (-13.2, 36.3)
  line L5956 (-13.2, 36.3) -> (-14.2, 36.3)
  line L5957 (-14.2, 36.3) -> (-14.2, 37.3)
  line L5958 (-14.2, 37.3) -> (-13.2, 37.3)
  line L5959 (-11.5, 39) -> (-11.5, 38)
  line L5960 (-11.5, 38) -> (-12.5, 38)
  line L5961 (-12.5, 38) -> (-12.5, 39)
  line L5962 (-12.5, 39) -> (-11.5, 39)
  line L5963 (-11.5, 37.2) -> (-11.5, 36.2)
  line L5964 (-11.5, 36.2) -> (-12.5, 36.2)
  line L5965 (-12.5, 36.2) -> (-12.5, 37.2)
  line L5966 (-12.5, 37.2) -> (-11.5, 37.2)
  line L5967 (-4.542, 13.47) -> (-5.542, 13.47)
  line L5968 (-5.542, 13.47) -> (-5.542, 14.47)
  line L5969 (-5.542, 14.47) -> (-4.542, 14.47)
  line L5970 (-4.542, 14.47) -> (-4.542, 13.47)
  line L5971 (-6.142, 13.47) -> (-7.142, 13.47)
  line L5972 (-7.142, 13.47) -> (-7.142, 14.47)
  line L5973 (-7.142, 14.47) -> (-6.142, 14.47)
  line L5974 (-6.142, 14.47) -> (-6.142, 13.47)
  line L5975 (-7.142, 20.058) -> (-6.142, 20.058)
  line L5976 (-6.142, 20.058) -> (-6.142, 19.058)
  line L5977 (-6.142, 19.058) -> (-7.142, 19.058)
  line L5978 (-7.142, 19.058) -> (-7.142, 20.058)
  line L5979 (-5.542, 20.058) -> (-4.542, 20.058)
  line L5980 (-4.542, 20.058) -> (-4.542, 19.058)
  line L5981 (-4.542, 19.058) -> (-5.542, 19.058)
  line L5982 (-5.542, 19.058) -> (-5.542, 20.058)
  line L5983 (-28.0642, 20.3777) -> (-28.7713, 19.6706)
  line L5984 (-28.7713, 19.6706) -> (-29.4784, 20.3777)
  line L5985 (-29.4784, 20.3777) -> (-28.7713, 21.0848)
  line L5986 (-28.7713, 21.0848) -> (-28.0642, 20.3777)
  line L5987 (-29.1956, 19.2463) -> (-29.9027, 18.5392)
  line L5988 (-29.9027, 18.5392) -> (-30.6098, 19.2463)
  line L5989 (-30.6098, 19.2463) -> (-29.9027, 19.9534)
  line L5990 (-29.9027, 19.9534) -> (-29.1956, 19.2463)
  line L5991 (-20.985, 6.977) -> (-19.985, 6.977)
  line L5992 (-19.985, 6.977) -> (-19.985, 5.977)
  line L5993 (-19.985, 5.977) -> (-20.985, 5.977)
  line L5994 (-20.985, 5.977) -> (-20.985, 6.977)
  line L5995 (-19.385, 6.977) -> (-18.385, 6.977)
  line L5996 (-18.385, 6.977) -> (-18.385, 5.977)
  line L5997 (-18.385, 5.977) -> (-19.385, 5.977)
  line L5998 (-19.385, 5.977) -> (-19.385, 6.977)
  line L5999 (-17.981, 1.829) -> (-18.981, 1.829)
  line L6000 (-18.981, 1.829) -> (-18.981, 2.829)
  line L6001 (-18.981, 2.829) -> (-17.981, 2.829)
  line L6002 (-17.981, 2.829) -> (-17.981, 1.829)
  line L6003 (-19.881, 1.829) -> (-20.881, 1.829)
  line L6004 (-20.881, 1.829) -> (-20.881, 2.829)
  line L6005 (-20.881, 2.829) -> (-19.881, 2.829)
  line L6006 (-19.881, 2.829) -> (-19.881, 1.829)
  line L6007 (-18.931, 4.029) -> (-19.931, 4.029)
  line L6008 (-19.931, 4.029) -> (-19.931, 5.029)
  line L6009 (-19.931, 5.029) -> (-18.931, 5.029)
  line L6010 (-18.931, 5.029) -> (-18.931, 4.029)
  circle A429 centre (-7.874, 6.096) radius 0.5
  circle A430 centre (-7.874, 43.053) radius 0.5
  circle A431 centre (-27.94, 43.053) radius 0.5
  circle A432 centre (-7.874, 6.096) radius 0.5
  circle A433 centre (-7.874, 43.053) radius 0.5
  circle A434 centre (-27.94, 43.053) radius 0.5
  circle A435 centre (-3.302, 41.148) radius 2.667
  circle A436 centre (-3.302, 41.148) radius 1.908
  circle A437 centre (-3.302, 41.148) radius 1.908
  circle A438 centre (-3.302, 41.148) radius 2.667
  circle A439 centre (-32.258, 41.148) radius 2.667
  circle A440 centre (-32.258, 41.148) radius 1.908
  circle A441 centre (-32.258, 41.148) radius 1.908
  circle A442 centre (-32.258, 41.148) radius 2.667
  line L6011 (-33.0454, 18.9463) -> (-33.0454, 19.6617)
  line L6012 (-33.0454, 19.6617) -> (-33.5513, 20.1676)
  line L6013 (-33.5513, 20.1676) -> (-34.2667, 20.1676)
  line L6014 (-34.2667, 20.1676) -> (-34.7726, 19.6617)
  line L6015 (-34.7726, 19.6617) -> (-34.7726, 18.9463)
  line L6016 (-34.7726, 18.9463) -> (-34.2667, 18.4404)
  line L6017 (-34.2667, 18.4404) -> (-33.5513, 18.4404)
  line L6018 (-33.5513, 18.4404) -> (-33.0454, 18.9463)
  circle A443 centre (-33.909, 19.304) radius 0.8636
  circle A444 centre (-33.909, 19.304) radius 0.8636
  line L6019 (-33.0454, 18.9463) -> (-33.0454, 19.6617)
  line L6020 (-33.0454, 19.6617) -> (-33.5513, 20.1676)
  line L6021 (-33.5513, 20.1676) -> (-34.2667, 20.1676)
  line L6022 (-34.2667, 20.1676) -> (-34.7726, 19.6617)
  line L6023 (-34.7726, 19.6617) -> (-34.7726, 18.9463)
  line L6024 (-34.7726, 18.9463) -> (-34.2667, 18.4404)
  line L6025 (-34.2667, 18.4404) -> (-33.5513, 18.4404)
  line L6026 (-33.5513, 18.4404) -> (-33.0454, 18.9463)
  line L6027 (-33.0454, 16.4063) -> (-33.0454, 17.1217)
  line L6028 (-33.0454, 17.1217) -> (-33.5513, 17.6276)
  line L6029 (-33.5513, 17.6276) -> (-34.2667, 17.6276)
  line L6030 (-34.2667, 17.6276) -> (-34.7726, 17.1217)
  line L6031 (-34.7726, 17.1217) -> (-34.7726, 16.4063)
  line L6032 (-34.7726, 16.4063) -> (-34.2667, 15.9004)
  line L6033 (-34.2667, 15.9004) -> (-33.5513, 15.9004)
  line L6034 (-33.5513, 15.9004) -> (-33.0454, 16.4063)
  circle A445 centre (-33.909, 16.764) radius 0.8636
  circle A446 centre (-33.909, 16.764) radius 0.8636
  line L6035 (-33.0454, 16.4063) -> (-33.0454, 17.1217)
  line L6036 (-33.0454, 17.1217) -> (-33.5513, 17.6276)
  line L6037 (-33.5513, 17.6276) -> (-34.2667, 17.6276)
  line L6038 (-34.2667, 17.6276) -> (-34.7726, 17.1217)
  line L6039 (-34.7726, 17.1217) -> (-34.7726, 16.4063)
  line L6040 (-34.7726, 16.4063) -> (-34.2667, 15.9004)
  line L6041 (-34.2667, 15.9004) -> (-33.5513, 15.9004)
  line L6042 (-33.5513, 15.9004) -> (-33.0454, 16.4063)
  line L6043 (-33.0454, 13.8663) -> (-33.0454, 14.5817)
  line L6044 (-33.0454, 14.5817) -> (-33.5513, 15.0876)
  line L6045 (-33.5513, 15.0876) -> (-34.2667, 15.0876)
  line L6046 (-34.2667, 15.0876) -> (-34.7726, 14.5817)
  line L6047 (-34.7726, 14.5817) -> (-34.7726, 13.8663)
  line L6048 (-34.7726, 13.8663) -> (-34.2667, 13.3604)
  line L6049 (-34.2667, 13.3604) -> (-33.5513, 13.3604)
  line L6050 (-33.5513, 13.3604) -> (-33.0454, 13.8663)
  circle A447 centre (-33.909, 14.224) radius 0.8636
  circle A448 centre (-33.909, 14.224) radius 0.8636
  line L6051 (-33.0454, 13.8663) -> (-33.0454, 14.5817)
  line L6052 (-33.0454, 14.5817) -> (-33.5513, 15.0876)
  line L6053 (-33.5513, 15.0876) -> (-34.2667, 15.0876)
  line L6054 (-34.2667, 15.0876) -> (-34.7726, 14.5817)
  line L6055 (-34.7726, 14.5817) -> (-34.7726, 13.8663)
  line L6056 (-34.7726, 13.8663) -> (-34.2667, 13.3604)
  line L6057 (-34.2667, 13.3604) -> (-33.5513, 13.3604)
  line L6058 (-33.5513, 13.3604) -> (-33.0454, 13.8663)
  line L6059 (-33.0454, 11.3263) -> (-33.0454, 12.0417)
  line L6060 (-33.0454, 12.0417) -> (-33.5513, 12.5476)
  line L6061 (-33.5513, 12.5476) -> (-34.2667, 12.5476)
  line L6062 (-34.2667, 12.5476) -> (-34.7726, 12.0417)
  line L6063 (-34.7726, 12.0417) -> (-34.7726, 11.3263)
  line L6064 (-34.7726, 11.3263) -> (-34.2667, 10.8204)
  line L6065 (-34.2667, 10.8204) -> (-33.5513, 10.8204)
  line L6066 (-33.5513, 10.8204) -> (-33.0454, 11.3263)
  circle A449 centre (-33.909, 11.684) radius 0.8636
  circle A450 centre (-33.909, 11.684) radius 0.8636
  line L6067 (-33.0454, 11.3263) -> (-33.0454, 12.0417)
  line L6068 (-33.0454, 12.0417) -> (-33.5513, 12.5476)
  line L6069 (-33.5513, 12.5476) -> (-34.2667, 12.5476)
  line L6070 (-34.2667, 12.5476) -> (-34.7726, 12.0417)
  line L6071 (-34.7726, 12.0417) -> (-34.7726, 11.3263)
  line L6072 (-34.7726, 11.3263) -> (-34.2667, 10.8204)
  line L6073 (-34.2667, 10.8204) -> (-33.5513, 10.8204)
  line L6074 (-33.5513, 10.8204) -> (-33.0454, 11.3263)
  line L6075 (-33.0454, 8.7863) -> (-33.0454, 9.5017)
  line L6076 (-33.0454, 9.5017) -> (-33.5513, 10.0076)
  line L6077 (-33.5513, 10.0076) -> (-34.2667, 10.0076)
  line L6078 (-34.2667, 10.0076) -> (-34.7726, 9.5017)
  line L6079 (-34.7726, 9.5017) -> (-34.7726, 8.7863)
  line L6080 (-34.7726, 8.7863) -> (-34.2667, 8.2804)
  line L6081 (-34.2667, 8.2804) -> (-33.5513, 8.2804)
  line L6082 (-33.5513, 8.2804) -> (-33.0454, 8.7863)
  circle A451 centre (-33.909, 9.144) radius 0.8636
  circle A452 centre (-33.909, 9.144) radius 0.8636
  line L6083 (-33.0454, 8.7863) -> (-33.0454, 9.5017)
  line L6084 (-33.0454, 9.5017) -> (-33.5513, 10.0076)
  line L6085 (-33.5513, 10.0076) -> (-34.2667, 10.0076)
  line L6086 (-34.2667, 10.0076) -> (-34.7726, 9.5017)
  line L6087 (-34.7726, 9.5017) -> (-34.7726, 8.7863)
  line L6088 (-34.7726, 8.7863) -> (-34.2667, 8.2804)
  line L6089 (-34.2667, 8.2804) -> (-33.5513, 8.2804)
  line L6090 (-33.5513, 8.2804) -> (-33.0454, 8.7863)
  line L6091 (-33.0454, 6.2463) -> (-33.0454, 6.9617)
  line L6092 (-33.0454, 6.9617) -> (-33.5513, 7.4676)
  line L6093 (-33.5513, 7.4676) -> (-34.2667, 7.4676)
  line L6094 (-34.2667, 7.4676) -> (-34.7726, 6.9617)
  line L6095 (-34.7726, 6.9617) -> (-34.7726, 6.2463)
  line L6096 (-34.7726, 6.2463) -> (-34.2667, 5.7404)
  line L6097 (-34.2667, 5.7404) -> (-33.5513, 5.7404)
  line L6098 (-33.5513, 5.7404) -> (-33.0454, 6.2463)
  circle A453 centre (-33.909, 6.604) radius 0.8636
  circle A454 centre (-33.909, 6.604) radius 0.8636
  line L6099 (-33.0454, 6.2463) -> (-33.0454, 6.9617)
  line L6100 (-33.0454, 6.9617) -> (-33.5513, 7.4676)
  line L6101 (-33.5513, 7.4676) -> (-34.2667, 7.4676)
  line L6102 (-34.2667, 7.4676) -> (-34.7726, 6.9617)
  line L6103 (-34.7726, 6.9617) -> (-34.7726, 6.2463)
  line L6104 (-34.7726, 6.2463) -> (-34.2667, 5.7404)
  line L6105 (-34.2667, 5.7404) -> (-33.5513, 5.7404)
  line L6106 (-33.5513, 5.7404) -> (-33.0454, 6.2463)
  line L6107 (-33.0454, 3.7063) -> (-33.0454, 4.4217)
  line L6108 (-33.0454, 4.4217) -> (-33.5513, 4.9276)
  line L6109 (-33.5513, 4.9276) -> (-34.2667, 4.9276)
  line L6110 (-34.2667, 4.9276) -> (-34.7726, 4.4217)
  line L6111 (-34.7726, 4.4217) -> (-34.7726, 3.7063)
  line L6112 (-34.7726, 3.7063) -> (-34.2667, 3.2004)
  line L6113 (-34.2667, 3.2004) -> (-33.5513, 3.2004)
  line L6114 (-33.5513, 3.2004) -> (-33.0454, 3.7063)
  circle A455 centre (-33.909, 4.064) radius 0.8636
  circle A456 centre (-33.909, 4.064) radius 0.8636
  line L6115 (-33.0454, 3.7063) -> (-33.0454, 4.4217)
  line L6116 (-33.0454, 4.4217) -> (-33.5513, 4.9276)
  line L6117 (-33.5513, 4.9276) -> (-34.2667, 4.9276)
  line L6118 (-34.2667, 4.9276) -> (-34.7726, 4.4217)
  line L6119 (-34.7726, 4.4217) -> (-34.7726, 3.7063)
  line L6120 (-34.7726, 3.7063) -> (-34.2667, 3.2004)
  line L6121 (-34.2667, 3.2004) -> (-33.5513, 3.2004)
  line L6122 (-33.5513, 3.2004) -> (-33.0454, 3.7063)
  line L6123 (-33.0454, 1.1663) -> (-33.0454, 1.8817)
  line L6124 (-33.0454, 1.8817) -> (-33.5513, 2.3876)
  line L6125 (-33.5513, 2.3876) -> (-34.2667, 2.3876)
  line L6126 (-34.2667, 2.3876) -> (-34.7726, 1.8817)
  line L6127 (-34.7726, 1.8817) -> (-34.7726, 1.1663)
  line L6128 (-34.7726, 1.1663) -> (-34.2667, 0.6604)
  line L6129 (-34.2667, 0.6604) -> (-33.5513, 0.6604)
  line L6130 (-33.5513, 0.6604) -> (-33.0454, 1.1663)
  circle A457 centre (-33.909, 1.524) radius 0.8636
  circle A458 centre (-33.909, 1.524) radius 0.8636
  line L6131 (-33.0454, 1.1663) -> (-33.0454, 1.8817)
  line L6132 (-33.0454, 1.8817) -> (-33.5513, 2.3876)
  line L6133 (-33.5513, 2.3876) -> (-34.2667, 2.3876)
  line L6134 (-34.2667, 2.3876) -> (-34.7726, 1.8817)
  line L6135 (-34.7726, 1.8817) -> (-34.7726, 1.1663)
  line L6136 (-34.7726, 1.1663) -> (-34.2667, 0.6604)
  line L6137 (-34.2667, 0.6604) -> (-33.5513, 0.6604)
  line L6138 (-33.5513, 0.6604) -> (-33.0454, 1.1663)
  line L6139 (-0.7874, 18.9463) -> (-0.7874, 19.6617)
  line L6140 (-0.7874, 19.6617) -> (-1.2933, 20.1676)
  line L6141 (-1.2933, 20.1676) -> (-2.0087, 20.1676)
  line L6142 (-2.0087, 20.1676) -> (-2.5146, 19.6617)
  line L6143 (-2.5146, 19.6617) -> (-2.5146, 18.9463)
  line L6144 (-2.5146, 18.9463) -> (-2.0087, 18.4404)
  line L6145 (-2.0087, 18.4404) -> (-1.2933, 18.4404)
  line L6146 (-1.2933, 18.4404) -> (-0.7874, 18.9463)
  circle A459 centre (-1.651, 19.304) radius 0.8636
  circle A460 centre (-1.651, 19.304) radius 0.8636
  line L6147 (-0.7874, 18.9463) -> (-0.7874, 19.6617)
  line L6148 (-0.7874, 19.6617) -> (-1.2933, 20.1676)
  line L6149 (-1.2933, 20.1676) -> (-2.0087, 20.1676)
  line L6150 (-2.0087, 20.1676) -> (-2.5146, 19.6617)
  line L6151 (-2.5146, 19.6617) -> (-2.5146, 18.9463)
  line L6152 (-2.5146, 18.9463) -> (-2.0087, 18.4404)
  line L6153 (-2.0087, 18.4404) -> (-1.2933, 18.4404)
  line L6154 (-1.2933, 18.4404) -> (-0.7874, 18.9463)
  line L6155 (-0.7874, 16.4063) -> (-0.7874, 17.1217)
  line L6156 (-0.7874, 17.1217) -> (-1.2933, 17.6276)
  line L6157 (-1.2933, 17.6276) -> (-2.0087, 17.6276)
  line L6158 (-2.0087, 17.6276) -> (-2.5146, 17.1217)
  line L6159 (-2.5146, 17.1217) -> (-2.5146, 16.4063)
  line L6160 (-2.5146, 16.4063) -> (-2.0087, 15.9004)
  line L6161 (-2.0087, 15.9004) -> (-1.2933, 15.9004)
  line L6162 (-1.2933, 15.9004) -> (-0.7874, 16.4063)
  circle A461 centre (-1.651, 16.764) radius 0.8636
  circle A462 centre (-1.651, 16.764) radius 0.8636
  line L6163 (-0.7874, 16.4063) -> (-0.7874, 17.1217)
  line L6164 (-0.7874, 17.1217) -> (-1.2933, 17.6276)
  line L6165 (-1.2933, 17.6276) -> (-2.0087, 17.6276)
  line L6166 (-2.0087, 17.6276) -> (-2.5146, 17.1217)
  line L6167 (-2.5146, 17.1217) -> (-2.5146, 16.4063)
  line L6168 (-2.5146, 16.4063) -> (-2.0087, 15.9004)
  line L6169 (-2.0087, 15.9004) -> (-1.2933, 15.9004)
  line L6170 (-1.2933, 15.9004) -> (-0.7874, 16.4063)
  line L6171 (-0.7874, 13.8663) -> (-0.7874, 14.5817)
  line L6172 (-0.7874, 14.5817) -> (-1.2933, 15.0876)
  line L6173 (-1.2933, 15.0876) -> (-2.0087, 15.0876)
  line L6174 (-2.0087, 15.0876) -> (-2.5146, 14.5817)
  line L6175 (-2.5146, 14.5817) -> (-2.5146, 13.8663)
  line L6176 (-2.5146, 13.8663) -> (-2.0087, 13.3604)
  line L6177 (-2.0087, 13.3604) -> (-1.2933, 13.3604)
  line L6178 (-1.2933, 13.3604) -> (-0.7874, 13.8663)
  circle A463 centre (-1.651, 14.224) radius 0.8636
  circle A464 centre (-1.651, 14.224) radius 0.8636
  line L6179 (-0.7874, 13.8663) -> (-0.7874, 14.5817)
  line L6180 (-0.7874, 14.5817) -> (-1.2933, 15.0876)
  line L6181 (-1.2933, 15.0876) -> (-2.0087, 15.0876)
  line L6182 (-2.0087, 15.0876) -> (-2.5146, 14.5817)
  line L6183 (-2.5146, 14.5817) -> (-2.5146, 13.8663)
  line L6184 (-2.5146, 13.8663) -> (-2.0087, 13.3604)
  line L6185 (-2.0087, 13.3604) -> (-1.2933, 13.3604)
  line L6186 (-1.2933, 13.3604) -> (-0.7874, 13.8663)
  line L6187 (-0.7874, 11.3263) -> (-0.7874, 12.0417)
  line L6188 (-0.7874, 12.0417) -> (-1.2933, 12.5476)
  line L6189 (-1.2933, 12.5476) -> (-2.0087, 12.5476)
  line L6190 (-2.0087, 12.5476) -> (-2.5146, 12.0417)
  line L6191 (-2.5146, 12.0417) -> (-2.5146, 11.3263)
  line L6192 (-2.5146, 11.3263) -> (-2.0087, 10.8204)
  line L6193 (-2.0087, 10.8204) -> (-1.2933, 10.8204)
  line L6194 (-1.2933, 10.8204) -> (-0.7874, 11.3263)
  circle A465 centre (-1.651, 11.684) radius 0.8636
  circle A466 centre (-1.651, 11.684) radius 0.8636
  line L6195 (-0.7874, 11.3263) -> (-0.7874, 12.0417)
  line L6196 (-0.7874, 12.0417) -> (-1.2933, 12.5476)
  line L6197 (-1.2933, 12.5476) -> (-2.0087, 12.5476)
  line L6198 (-2.0087, 12.5476) -> (-2.5146, 12.0417)
  line L6199 (-2.5146, 12.0417) -> (-2.5146, 11.3263)
  line L6200 (-2.5146, 11.3263) -> (-2.0087, 10.8204)
  line L6201 (-2.0087, 10.8204) -> (-1.2933, 10.8204)
  line L6202 (-1.2933, 10.8204) -> (-0.7874, 11.3263)
  line L6203 (-0.7874, 8.7863) -> (-0.7874, 9.5017)
  line L6204 (-0.7874, 9.5017) -> (-1.2933, 10.0076)
  line L6205 (-1.2933, 10.0076) -> (-2.0087, 10.0076)
  line L6206 (-2.0087, 10.0076) -> (-2.5146, 9.5017)
  line L6207 (-2.5146, 9.5017) -> (-2.5146, 8.7863)
  line L6208 (-2.5146, 8.7863) -> (-2.0087, 8.2804)
  line L6209 (-2.0087, 8.2804) -> (-1.2933, 8.2804)
  line L6210 (-1.2933, 8.2804) -> (-0.7874, 8.7863)
  circle A467 centre (-1.651, 9.144) radius 0.8636
  circle A468 centre (-1.651, 9.144) radius 0.8636
  line L6211 (-0.7874, 8.7863) -> (-0.7874, 9.5017)
  line L6212 (-0.7874, 9.5017) -> (-1.2933, 10.0076)
  line L6213 (-1.2933, 10.0076) -> (-2.0087, 10.0076)
  line L6214 (-2.0087, 10.0076) -> (-2.5146, 9.5017)
  line L6215 (-2.5146, 9.5017) -> (-2.5146, 8.7863)
  line L6216 (-2.5146, 8.7863) -> (-2.0087, 8.2804)
  line L6217 (-2.0087, 8.2804) -> (-1.2933, 8.2804)
  line L6218 (-1.2933, 8.2804) -> (-0.7874, 8.7863)
  line L6219 (-0.7874, 6.2463) -> (-0.7874, 6.9617)
  line L6220 (-0.7874, 6.9617) -> (-1.2933, 7.4676)
  line L6221 (-1.2933, 7.4676) -> (-2.0087, 7.4676)
  line L6222 (-2.0087, 7.4676) -> (-2.5146, 6.9617)
  line L6223 (-2.5146, 6.9617) -> (-2.5146, 6.2463)
  line L6224 (-2.5146, 6.2463) -> (-2.0087, 5.7404)
  line L6225 (-2.0087, 5.7404) -> (-1.2933, 5.7404)
  line L6226 (-1.2933, 5.7404) -> (-0.7874, 6.2463)
  circle A469 centre (-1.651, 6.604) radius 0.8636
  circle A470 centre (-1.651, 6.604) radius 0.8636
  line L6227 (-0.7874, 6.2463) -> (-0.7874, 6.9617)
  line L6228 (-0.7874, 6.9617) -> (-1.2933, 7.4676)
  line L6229 (-1.2933, 7.4676) -> (-2.0087, 7.4676)
  line L6230 (-2.0087, 7.4676) -> (-2.5146, 6.9617)
  line L6231 (-2.5146, 6.9617) -> (-2.5146, 6.2463)
  line L6232 (-2.5146, 6.2463) -> (-2.0087, 5.7404)
  line L6233 (-2.0087, 5.7404) -> (-1.2933, 5.7404)
  line L6234 (-1.2933, 5.7404) -> (-0.7874, 6.2463)
  line L6235 (-0.7874, 3.7063) -> (-0.7874, 4.4217)
  line L6236 (-0.7874, 4.4217) -> (-1.2933, 4.9276)
  line L6237 (-1.2933, 4.9276) -> (-2.0087, 4.9276)
  line L6238 (-2.0087, 4.9276) -> (-2.5146, 4.4217)
  line L6239 (-2.5146, 4.4217) -> (-2.5146, 3.7063)
  line L6240 (-2.5146, 3.7063) -> (-2.0087, 3.2004)
  line L6241 (-2.0087, 3.2004) -> (-1.2933, 3.2004)
  line L6242 (-1.2933, 3.2004) -> (-0.7874, 3.7063)
  circle A471 centre (-1.651, 4.064) radius 0.8636
  circle A472 centre (-1.651, 4.064) radius 0.8636
  line L6243 (-0.7874, 3.7063) -> (-0.7874, 4.4217)
  line L6244 (-0.7874, 4.4217) -> (-1.2933, 4.9276)
  line L6245 (-1.2933, 4.9276) -> (-2.0087, 4.9276)
  line L6246 (-2.0087, 4.9276) -> (-2.5146, 4.4217)
  line L6247 (-2.5146, 4.4217) -> (-2.5146, 3.7063)
  line L6248 (-2.5146, 3.7063) -> (-2.0087, 3.2004)
  line L6249 (-2.0087, 3.2004) -> (-1.2933, 3.2004)
  line L6250 (-1.2933, 3.2004) -> (-0.7874, 3.7063)
  line L6251 (-0.7874, 1.1663) -> (-0.7874, 1.8817)
  line L6252 (-0.7874, 1.8817) -> (-1.2933, 2.3876)
  line L6253 (-1.2933, 2.3876) -> (-2.0087, 2.3876)
  line L6254 (-2.0087, 2.3876) -> (-2.5146, 1.8817)
  line L6255 (-2.5146, 1.8817) -> (-2.5146, 1.1663)
  line L6256 (-2.5146, 1.1663) -> (-2.0087, 0.6604)
  line L6257 (-2.0087, 0.6604) -> (-1.2933, 0.6604)
  line L6258 (-1.2933, 0.6604) -> (-0.7874, 1.1663)
  circle A473 centre (-1.651, 1.524) radius 0.8636
  circle A474 centre (-1.651, 1.524) radius 0.8636
  line L6259 (-0.7874, 1.1663) -> (-0.7874, 1.8817)
  line L6260 (-0.7874, 1.8817) -> (-1.2933, 2.3876)
  line L6261 (-1.2933, 2.3876) -> (-2.0087, 2.3876)
  line L6262 (-2.0087, 2.3876) -> (-2.5146, 1.8817)
  line L6263 (-2.5146, 1.8817) -> (-2.5146, 1.1663)
  line L6264 (-2.5146, 1.1663) -> (-2.0087, 0.6604)
  line L6265 (-2.0087, 0.6604) -> (-1.2933, 0.6604)
  line L6266 (-1.2933, 0.6604) -> (-0.7874, 1.1663)
  line L6267 (-29.2354, 16.4063) -> (-29.2354, 17.1217)